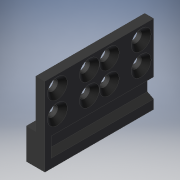
# Autodesk Inventor part: Montageplatte_R
Saved by Autodesk Inventor 2019 (Build 230136000, 136)
## iProperties
Created: 2022-03-19
Part Number: Montageplatte_R
Material: Generic
Document SubType Name: Modeling
Designer: Lukas
Density: 1 g/cm^3
Appearance: Default
Author: Lukas
Autodesk Inventor part; units mm, degrees
ref_plane "YZ Plane" through (0, 0, 0) normal (1, 0, 0) x (0, 1, 0)
ref_plane "XZ Plane" through (0, 0, 0) normal (0, 1, 0) x (-1, 0, 0)
ref_plane "XY Plane" through (0, 0, 0) normal (0, 0, 1) x (1, 0, 0)
sketch "Sketch1" plane through (0, 0, 0) normal (0, 0, 1) x (1, 0, 0)
  line L0 (0.1, 4.8) -> (-2.9, 4.8)
  line L1 (-2.9, 4.8) -> (-2.9, -4.8)
  line L2 (-2.9, -4.8) -> (2.9, -4.8)
  line L3 (2.9, -4.8) -> (2.9, 19.8)
  line L4 (2.9, 19.8) -> (0.1, 19.8)
  line L5 (0.1, 19.8) -> (0.1, 4.8)
  point P0 (0, 0)
  point P1 (0, -4.8)
  point P2 (-2.9, 0)
  dimension "d0" = 15
  dimension "d1" = 9.6
  dimension "d2" = 5.8
  dimension "d3" = 2.8
  constraints: 12 end point, 4 perpendicular, 2 midpoint, 1 horizontal, 1 horizontal alignment, 1 parallel, 1 vertical alignment
  measures "d0" distance of L4.end L0.start
  measures "d1" distance of L0.end L1.end
  measures "d2" distance of L1.end L2.end
  measures "d3" distance of L3.end L4.end
extrude "Extrusion1" add sketch "Sketch1" along normal blind 34
sketch "Sketch2" plane through (2.9, -4.8, 0) normal (1, 0, 0) x (0, 0, -1)
  circle A0 centre (-3.9, 13.8) radius 1.6
  circle A1 centre (-3.9, 20.8) radius 1.6
  circle A2 centre (-13.9, 13.8) radius 1.6
  circle A3 centre (-13.9, 20.8) radius 1.6
  circle A4 centre (-20.1, 13.8) radius 1.6
  circle A5 centre (-20.1, 20.8) radius 1.6
  circle A6 centre (-30.1, 20.8) radius 1.6
  circle A7 centre (-30.1, 13.8) radius 1.6
  line L0 (0, 24.6) -> (-34, 24.6) projected
  point P0 (0, 4.8)
  point P1 (-17, 17.3)
  point P2 (-17, 24.6)
  dimension "d6" = 3.8
  dimension "d7" = 10
  dimension "d8" = 6.2
  dimension "d9" = 10
  dimension "d10" = 3.1
  dimension "d11" = 7
  dimension "d12" = 3.5
  dimension "d13" = 3.2
  constraints: 8 centre point, 7 equal radius, 6 horizontal alignment, 5 vertical alignment, 1 midpoint
  measures "d6" distance from line of L0 A1.centre
  measures "d7" distance of A3.centre A1.centre
  measures "d8" distance of A5.centre A3.centre
  measures "d9" distance of A6.centre A5.centre
  measures "d10" horizontal distance of A3.centre point (-17, 17.3)
  measures "d11" distance of A0.centre A1.centre
  measures "d12" vertical distance of A2.centre point (-17, 17.3)
  measures "d13" diameter of A0
extrude "Extrusion2" cut sketch "Sketch2" against normal through all
chamfer "Chamfer1" distance 1.5 angle 45 8 edges at (2.9, 9, 5.5) (2.9, 9, 15.5) (2.9, 9, 21.7) (2.9, 9, 31.7) (2.9, 16, 31.7) (2.9, 16, 21.7) (2.9, 16, 15.5) (2.9, 16, 5.5)
sketch "Sketch3" plane through (0, 0, 0) normal (0, 0, -1) x (-1, 0, 0)
  line L0 (2.9, -4.8) -> (-2.9, -4.8) projected
  line L1 (-2.9, -4.8) -> (-2.9, 19.8) projected
  line L2 (-2.9, 4) -> (-0.9, 3)
  line L3 (-0.9, 3) -> (-0.9, -1)
  line L4 (-0.9, -1) -> (-2.9, -2)
  line L5 (-2.9, -2) -> (-2.9, 4)
  point P0 (0, 0)
  point P1 (-2.9, 1)
  point P2 (-0.9, 1)
  dimension "d25" = 2.8
  dimension "d26" = 6
  dimension "d27" = 4
  dimension "d28" = 2
  constraints: 8 end point, 2 midpoint, 2 parallel, 2 point on line, 1 horizontal alignment
  measures "d25" distance of L0.end L4.end
  measures "d26" distance of L4.end L2.start
  measures "d27" distance of L2.end L3.end
  measures "d28" distance between parallel lines of L5 L3
extrude "Extrusion3" cut sketch "Sketch3" against normal blind 32
equation "\"d10\" = 0.5 * d8"
equation "\"d12\" = 0.5 * d11"
body "Solid1"
